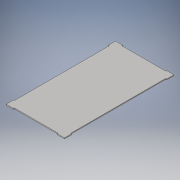
# Autodesk Inventor part: bottom
Saved by Autodesk Inventor 2016 SP2 (Build 200236200, 236)
## iProperties
Created: 2017-09-04
Part Number: bottom
Material: Generic
Document SubType Name: Modeling
Designer: Kartikye
Density: 1 g/cm^3
Appearance: Default
Author: Kartikye
Autodesk Inventor part; units mm, degrees
ref_plane "YZ Plane" through (0, 0, 0) normal (1, 0, 0) x (0, 1, 0)
ref_plane "XZ Plane" through (0, 0, 0) normal (0, 1, 0) x (-1, 0, 0)
ref_plane "XY Plane" through (0, 0, 0) normal (0, 0, 1) x (1, 0, 0)
sketch "Sketch1" plane through (0, 0, 0) normal (0, 1, 0) x (-1, 0, 0)
  line L0 (-101.6, 190.5) -> (101.6, 190.5)
  line L1 (101.6, 190.5) -> (101.6, -190.5)
  line L2 (101.6, -190.5) -> (-101.6, -190.5)
  line L3 (-101.6, -190.5) -> (-101.6, 190.5)
  line L4 (-101.6, 190.5) -> (101.6, -190.5) construction
  line L5 (101.6, 190.5) -> (-101.6, -190.5) construction
  point P0 (0, 0)
  dimension "d0" = 203.2
  dimension "d1" = 381
  constraints: 12 end point, 2 midpoint, 2 parallel, 1 horizontal, 1 perpendicular
  measures "d0" distance of L1.end L2.end
  measures "d1" distance of L0.end L1.end
extrude "Extrusion1" add sketch "Sketch1" along normal blind 3.175
sketch "Sketch2" plane through (0, 3.175, 0) normal (0, 1, 0) x (1, 0, 0)
  line L0 (-76.2, -190.5) -> (-76.2, -187.325)
  line L1 (-101.6, -165.1) -> (-98.425, -165.1)
  line L2 (-98.425, -165.1) -> (-98.425, 0)
  line L3 (-76.2, -187.325) -> (0, -187.325)
  line L4 (-101.6, 190.5) -> (-101.6, 165.1)
  line L5 (-101.6, 165.1) -> (-98.425, 165.1)
  line L6 (-98.425, 165.1) -> (-98.425, 0)
  line L7 (-101.6, 190.5) -> (-76.2, 190.5)
  line L8 (0, -187.325) -> (76.2, -187.325)
  line L9 (76.2, -187.325) -> (76.2, -190.5)
  line L10 (101.6, -190.5) -> (101.6, -165.1)
  line L11 (101.6, -190.5) -> (101.6, 190.5) projected
  line L12 (101.6, -165.1) -> (98.425, -165.1)
  line L13 (98.425, -165.1) -> (98.425, 165.1)
  line L14 (98.425, 165.1) -> (101.6, 165.1)
  line L15 (-76.2, 190.5) -> (-76.2, 187.325)
  line L16 (-76.2, 187.325) -> (76.2, 187.325)
  line L17 (76.2, 187.325) -> (76.2, 190.5)
  line L18 (76.2, 190.5) -> (-76.2, 190.5)
  line L19 (101.6, -165.1) -> (142.875, -125.4125)
  line L20 (142.875, -125.4125) -> (138.1125, 114.3)
  line L21 (138.1125, 114.3) -> (101.6, 165.1)
  line L22 (-76.2, -190.5) -> (66.675, -207.9625)
  line L23 (66.675, -207.9625) -> (76.2, -190.5)
  line L24 (-101.6, -165.1) -> (-173.0375, -100.0125)
  line L25 (-173.0375, -100.0125) -> (-152.4, 165.1)
  line L26 (-152.4, 165.1) -> (-101.6, 165.1)
  point P0 (-101.6, -190.5)
  dimension "d5" = 25.4
  dimension "d6" = 76.2
  dimension "d7" = 180
  constraints: 53 end point, 6 perpendicular, 4 horizontal, 3 vertical, 2 point on line
  measures "d5" distance of point (-101.6, -190.5) L0.start
  measures "d6" distance of L3.end L8.end
  measures "d7" angle of L8 L3
extrude "Extrusion2" cut sketch "Sketch2" against normal blind 3.175 contours L0 L3 L8 L9 L23 L22 | L24 L25 L26 L5 L6 L2 L1 | L18 L17 L16 L15 | L12 L13 L14 L11
body "Solid1"
